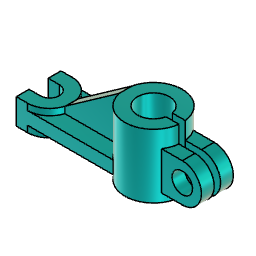
Design 7 v2 (Autodesk Fusion 360 design; units mm, degrees)
Autodesk Fusion 360 part; units mm, degrees
sketch "Sketch1" plane through (0, 0, 0) normal (0, 0, 1) x (1, 0, 0)
  line L0 (308.5786, -175) -> (-450, -175)
  line L1 (-450, 175) -> (308.5786, 175)
  line L2 (-362.5803, 75) -> (-450, 75)
  line L3 (-450, -75) -> (-362.5803, -75)
  line L4 (572.4745, -25) -> (673.6068, -25)
  line L5 (673.6068, 25) -> (572.4745, 25)
  line L6 (-194.8752, -50) -> (230.6259, -50)
  line L7 (230.6259, 50) -> (-190.6515, 50)
  arc A0 (-362.5803, -175) -> (-362.5803, 175) centre (-362.5803, 0) ccw
  arc A1 (-362.5803, -75) -> (-362.5803, 75) centre (-362.5803, 0) ccw
  line L8 (-450, -175) -> (-450, -75)
  line L9 (-450, 75) -> (-450, 175)
  line L10 (-187.5803, 0) -> (-287.5803, 0) construction
  line L11 (-437.5803, 0) -> (-450, 0) construction
  line L12 (0, 0) -> (251.3485, 0)
  line L13 (-190.6515, 50) -> (-193.5791, 45.4268)
  arc A2 (673.6068, 25) -> (674.4966, -15.0423) centre (450, 0) ccw
  arc A3 (573.9211, 16.3875) -> (573.9211, -16.3875) centre (450, 0) ccw
  dimension "d2" = 350
  dimension "d3" = 150
  dimension "d4" = 350
  dimension "d5" = 250
  dimension "d6" = 450
  dimension "d8" = 150
  constraint horizontal L0
  constraint perpendicular L0 L8
  constraint parallel L0 L1
  constraint perpendicular L8 L10
  constraint parallel L10 L12
  constraint concentric A0 A1
  constraint concentric A2 A3
  constraint horizontal L2
  constraint horizontal L3
  constraint horizontal L4
  constraint parallel L4 L5
  constraint horizontal L6
  constraint parallel L6 L7
  constraint coincident origin L12
  constraint coincident L2.end L8
  constraint coincident L11.start L10
  constraint collinear L8 L9
  constraint collinear L10 L11
  constraint coincident A1 L10.end
  constraint coincident L0 A0.start
  constraint coincident L6.end A2
  constraint coincident L7.start A2
  constraint coincident A0 L13.end
  constraint coincident A0 L6.start
  constraint coincident L4.end A2
  constraint coincident A3 L5.end
  constraint coincident A3 L4.start
  constraint coincident A2 L0.start
  constraint coincident A2 L1.end
  constraint coincident A0 L10.start
  constraint coincident L1 A0.end
  measures "d2" distance of L0.end L1.start
  measures "d3" diameter of A1
  measures "d4" diameter of A0
  measures "d5" diameter of A3
  measures "d6" diameter of A2
  measures "d8" distance of L2.start L3.end
extrude "Extrude1" add sketch "Sketch1" along normal mid plane 100 contours L0 L6 A0 A2 | L6 L7 A0 L13 A2 | L1 L7 A0 L13 A2 makes body 1
extrude "Extrude2" add sketch "Sketch1" along normal mid plane 200 contours L0 L1 L2 L3 A0 A1 L8 L9 bodies 1
extrude "Extrude3" add sketch "Sketch1" along normal blind 400 and the other way blind 100 contours L4 L5 A2 A3 bodies 1
extrude "Extrude4" add sketch "Sketch1" along normal blind 400 contours L6 L7 A0 L13 A2 bodies 1
sketch "Sketch2" plane through (0, -50, 0) normal (0, -1, 0) x (1, 0, 0)
  line L0 (-194.8752, 50) -> (230.6259, 50)
  line L1 (230.6259, 50) -> (230.6259, 400)
  line L2 (230.6259, 400) -> (-194.8752, 400)
  line L3 (-194.8752, 400) -> (-194.8752, 100)
  line L4 (-194.8752, 100) -> (-194.8752, 50)
  line L5 (230.6259, 400) -> (-194.8752, 100)
  line L6 (-194.8752, 100) -> (-194.8752, 400)
  line L7 (230.6259, 400) -> (-194.8752, 400)
  constraint coincident L1.end L2.start
  constraint coincident L3.end L4.start
  constraint coincident L2.end L3.start
extrude "Extrude5" cut sketch "Sketch2" against normal blind 450 contours L2 L3 L5 L6 L7 bodies 1
sketch "Sketch3" plane through (0, -50, 0) normal (0, -1, 0) x (1, 0, 0)
  line L0 (230.6259, 400) -> (-194.8752, 100)
  line L1 (-194.8752, 100) -> (-194.8752, 50)
  line L2 (-194.8752, 50) -> (230.6259, 50)
  line L3 (230.6259, 50) -> (230.6259, 400)
  circle A0 centre (800, 115.696) radius 80
  line L4 (800, 265.696) -> (410, 265.696)
  line L5 (410, 265.696) -> (410, -34.304)
  line L6 (410, -34.304) -> (800, -34.304)
  line L7 (800, -34.304) -> (800, 265.696)
  arc A1 (800, -34.304) -> (800, 265.696) centre (800, 115.696) ccw
  point P0 (-450, -100)
  point P1 (673.6068, -100)
  dimension "d25" = 160
  dimension "d26" = 300
  dimension "d27" = 390
  dimension "d28" = 300
  dimension "d29" = 1250
  dimension "d30" = 250
  constraint concentric A0 A1
  constraint horizontal L4
  constraint vertical L5
  constraint horizontal L6
  constraint vertical L7
  measures "d25" diameter of A0
  measures "d26" diameter of A1
  measures "d27" distance of L4.start L4.end
  measures "d28" distance of L4.start L6.end
  measures "d29" horizontal distance of A0.centre P0
  measures "d30" distance of A0.centre P1
extrude "Extrude6" add sketch "Sketch3" along normal blind 100 from surface at -25 separate body contours A0 L7 A1 | A0 L4 L5 L6 L7 makes body 2
combine "Combine1" operation cut target body 2 tool bodies 1 keep tools makes body 3 at (554.6904, -68.3002, 65.696)
delete_body "RemoveBody1" bodies 3
mirror "Mirror1" about plane through (0, 0, 0) normal (0, 1, 0) of bodies 2 makes body 4
